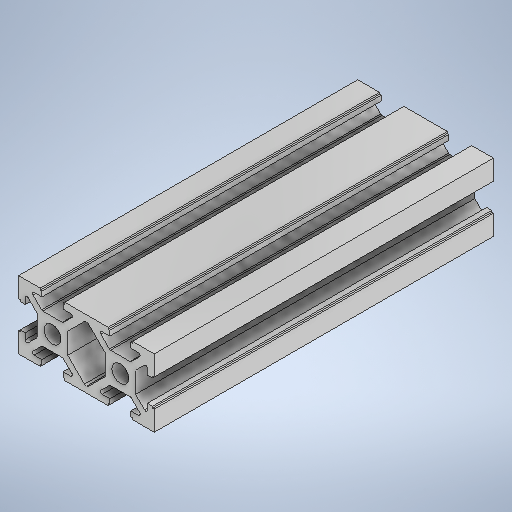
# Autodesk Inventor part: Perfil 20×40 6 rasgos_001
Saved by Autodesk Inventor 2026 (Build 300175000, 175)
## iProperties
Created: 2025-03-26
Part Number: Perfil 20×40 6 rasgos_001
Material: Generic
Document SubType Name: Modeling
Designer: Carlos Dias
Density: 1 g/cm^3
Appearance: Default
Author: Carlos Dias
Autodesk Inventor part; units mm, degrees
ref_plane "YZ Plane" through (0, 0, 0) normal (1, 0, 0) x (0, 1, 0)
ref_plane "XZ Plane" through (0, 0, 0) normal (0, 1, 0) x (-1, 0, 0)
ref_plane "XY Plane" through (0, 0, 0) normal (0, 0, 1) x (1, 0, 0)
sketch "Sketch1" plane through (0, 0, 0) normal (0, 0, 1) x (1, 0, 0)
  line L0 (0, 10) -> (0, -10) construction
  line L1 (-20, 10) -> (0, 10) construction
  line L2 (-10, 0) -> (0, 0) construction
  circle A0 centre (-10, 0) radius 2.5 construction
  line L3 (-13.1, 10) -> (-6.9, 10) construction
  line L4 (-14.5, 4.5) -> (-5.5, 4.5) construction
  line L5 (-5.5, 4.5) -> (-5.5, -4.5) construction
  line L6 (-14.5, -4.5) -> (-5.5, -4.5) construction
  line L7 (-14.5, 4.5) -> (-14.5, -4.5) construction
  line L8 (-20, -10) -> (0, 10) construction
  line L9 (-3.4142, 8) -> (-6.9142, 4.5) construction
  line L10 (-0.5858, 8) -> (-5.5, 3.0858)
  arc A1 (-7.5, 0) -> (-12.5, 0) centre (-10, 0) ccw
  line L11 (-5.5, 3.0858) -> (-5.5, 0)
  line L12 (-5.5, 0) -> (-7.5, 0)
  arc A2 (0, 8.255) -> (-0.5858, 8) centre (0.0312, 7.383) ccw
  line L13 (-6.9, 8) -> (-3.4142, 8) construction
  line L14 (-6.9, 10) -> (-6.9, 8) construction
  line L15 (-6.9, 10) -> (-6.4, 10) construction
  line L16 (-6.4, 10) -> (-6.4, 9.5)
  line L17 (-6.4, 9.5) -> (-6.9, 9.5)
  line L18 (-6.9, 9.5) -> (-6.9, 10) construction
  line L19 (-6.9, 9.5) -> (-6.9, 8)
  line L20 (-6.4, 10) -> (0, 10)
  line L21 (0, 10) -> (0, 8.255)
  line L22 (-20, 10) -> (0, -10) construction
  line L23 (-16.5858, 8) -> (-13.0858, 4.5) construction
  line L24 (-16.5858, 8) -> (-13.1, 8) construction
  line L25 (-13.1, 8) -> (-13.1, 10) construction
  line L26 (-13.1, 10) -> (-13.6, 10) construction
  line L27 (-13.6, 10) -> (-13.6, 9.5)
  line L28 (-13.6, 9.5) -> (-13.1, 9.5)
  line L29 (-13.1, 9.5) -> (-13.1, 10) construction
  line L30 (-13.1, 9.5) -> (-13.1, 8)
  line L31 (-13.6, 10) -> (-20, 10)
  line L32 (-20, 10) -> (-20, 3.6) construction
  line L33 (-20, 3.6) -> (-18, 3.6) construction
  line L34 (-18, 6.5858) -> (-14.5, 3.0858) construction
  line L35 (-18, 6.5858) -> (-18, 3.6) construction
  line L36 (-20, 3.6) -> (-19.5, 3.6) construction
  line L37 (-19.5, 3.6) -> (-19.5, 4.1)
  line L38 (-19.5, 4.1) -> (-20, 4.1)
  line L39 (-20, 4.1) -> (-20, 3.6) construction
  arc A3 (-13.2322, 4.6464) -> (-12.8787, 4.5) centre (-12.8787, 5) ccw
  arc A4 (-7.1213, 4.5) -> (-6.7678, 4.6464) centre (-7.1213, 5) ccw
  arc A5 (-17.1464, 5.7322) -> (-18, 5.3787) centre (-17.5, 5.3787) ccw
  arc A6 (-15.3787, 8) -> (-15.7322, 7.1464) centre (-15.3787, 7.5) ccw
  arc A7 (-4.2678, 7.1464) -> (-4.6213, 8) centre (-4.6213, 7.5) ccw
  line L40 (-12.8787, 4.5) -> (-7.1213, 4.5)
  line L41 (-15.7322, 7.1464) -> (-13.2322, 4.6464)
  line L42 (-15.3787, 8) -> (-13.1, 8)
  line L43 (-4.2678, 7.1464) -> (-6.7678, 4.6464)
  line L44 (-4.6213, 8) -> (-6.9, 8)
  line L45 (-14.5, 3.0858) -> (-17.1464, 5.7322)
  line L46 (-18, 3.6) -> (-19.5, 3.6)
  line L47 (-20, 10) -> (-20, 4.1)
  line L48 (-18, 5.3787) -> (-18, 3.6)
  line L49 (-14.5, 3.0858) -> (-14.5, 0)
  line L50 (-14.5, 0) -> (-12.5, 0)
  point P0 (-10, 10)
  point P1 (-10, 10)
  point P2 (-10, 4.5)
  point P3 (-10, -4.5)
  point P4 (-0.3171, 8.183)
  point P5 (-6.9, 9)
  point P6 (-14.5, 0)
  dimension "d5" = 5
  dimension "d0" = 20
  dimension "d1" = 20
  dimension "d4" = 10
  dimension "d6" = 6.2
  dimension "d8" = 2
  dimension "d9" = 1
  dimension "d10" = 1
  dimension "d11" = 2
  dimension "d12" = 2
  dimension "d13" = 0.8
  dimension "d14" = 0.5
  dimension "d16" = 1
  dimension "d17" = 0.5
  dimension "d18" = 6.4
  dimension "d20" = 1
  dimension "d21" = 0.5
  dimension "d22" = 0.5
  dimension "d23" = 0.5
  dimension "d24" = 0.5
  dimension "d25" = 0.5
  dimension "d26" = 0.5
  constraints: 102 end point, 18 point on line, 16 point on circle, 14 horizontal, 11 tangent, 10 collinear, 10 midpoint, 9 parallel, 8 vertical, 7 centre point, 7 equal length, 5 coincident, 5 horizontal alignment, 5 vertical alignment, 3 perpendicular, 2 other
  measures "d0" distance of L0.start L0.end
  measures "d1" distance of L0.start L1.start
  measures "d4" distance of L2.start L2.end
  measures "d6" distance of L3.start L3.end
  measures "d9" distance between parallel lines of L8 L9
  measures "d10" distance between parallel lines of L8 L10
  measures "d11" distance from line of L9.start L1
  measures "d12" distance from line of L10.start L1
  measures "d13" vertical distance of A2.centre point (-0.317, 8.183)
  measures "d14" distance of L16.end L17.end
  measures "d16" distance between parallel lines of L22 L23
  measures "d17" distance of L27.end L28.end
  measures "d18" distance of L1.start L32.end
  measures "d20" distance between parallel lines of L22 L34
  measures "d21" distance of L37.end L38.end
  measures "d22" radius of A3
  measures "d23" radius of A4
  measures "d24" radius of A5
  measures "d25" radius of A6
  measures "d26" radius of A7
extrude "Extrusion1" add sketch "Sketch1" along normal mid plane 100
mirror "Mirror1" about plane through (0, 0, 0) normal (0, 1, 0) of "Extrusion1"
mirror "Mirror2" about plane through (0, 0, 0) normal (1, 0, 0) of "Extrusion1", "Mirror1"
equation "\"d10\" = d9"
equation "\"d16\" = d9"
equation "\"d17\" = d14"
equation "\"d20\" = d9"
equation "\"d21\" = d14"
equation "\"d23\" = d22"
equation "\"d24\" = d22"
equation "\"d25\" = d22"
equation "\"d26\" = d22"
body "Solid1"
